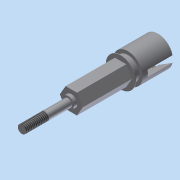
# Autodesk Inventor part: Shaft
Saved by Autodesk Inventor 2011 SP1 (Build 150282100, 282)
## iProperties
Created: 2011-09-20
Part Number: Shaft
Document SubType Name: Modeling
Designer: dgitz
Density: 1 g/cm^3
Author: dgitz
Autodesk Inventor part; units mm, degrees
ref_plane "YZ Plane" through (0, 0, 0) normal (1, 0, 0) x (0, 1, 0)
ref_plane "XZ Plane" through (0, 0, 0) normal (0, 1, 0) x (-1, 0, 0)
ref_plane "XY Plane" through (0, 0, 0) normal (0, 0, 1) x (1, 0, 0)
sketch "Sketch1" plane through (0, 0, 0) normal (0, 0, 1) x (1, 0, 0)
  line L0 (2.1997, -3.81) -> (-2.1997, -3.81)
  line L1 (-2.1997, -3.81) -> (-4.3994, 0)
  line L2 (-4.3994, 0) -> (-2.1997, 3.81)
  line L3 (-2.1997, 3.81) -> (2.1997, 3.81)
  line L4 (2.1997, 3.81) -> (4.3994, 0)
  line L5 (4.3994, 0) -> (2.1997, -3.81)
  point P0 (0, 0)
  point P1 (0, 0)
  dimension "d0" = 7.62
  constraints: 12 end point, 1 coincident, 1 horizontal, 13 other
  measures "d0" distance between parallel lines of L0 L3
extrude "Extrusion1" add sketch "Sketch1" along normal blind 19.05
sketch "Sketch2" plane through (0, 0, 19.05) normal (0, 0, 1) x (1, 0, 0)
  circle A0 centre (0, 0) radius 2.286
  dimension "d3" = 4.572
  constraints: 1 centre point, 1 coincident
  measures "d3" diameter of A0
extrude "Extrusion2" add sketch "Sketch2" along normal blind 1.27
sketch "Sketch3" plane through (0, 0, 20.32) normal (0, 0, 1) x (1, 0, 0)
  circle A0 centre (0, 0) radius 2.286 projected
  circle A1 centre (0, 0) radius 1.5875
  dimension "d6" = 3.175
  constraints: 1 centre point, 1 coincident
  measures "d6" diameter of A1
extrude "Extrusion3" add sketch "Sketch3" along normal blind 17.78 contours A1
thread "Thread1" size "5-40 UNC" class "2A" standard "ANSI Unified Screw Threads" length 8.89
sketch "Sketch4" plane through (0, 0, 0) normal (0, 0, -1) x (-1, 0, 0)
  circle A0 centre (0, 0) radius 5.715
  dimension "d11" = 11.43
  constraints: 1 centre point, 1 coincident
  measures "d11" diameter of A0
extrude "Extrusion4" add sketch "Sketch4" along normal blind 0.254
sketch "Sketch5" plane through (0, 0, -0.254) normal (0, 0, -1) x (-1, 0, 0)
  circle A0 centre (0, 0) radius 5.715 projected
  circle A1 centre (0, 0) radius 4.445
  dimension "d14" = 8.89
  constraints: 1 centre point, 1 coincident
  measures "d14" diameter of A1
extrude "Extrusion5" add sketch "Sketch5" along normal blind 2.54 contours A1
sketch "Sketch6" plane through (0, 0, -2.794) normal (0, 0, -1) x (-1, 0, 0)
  circle A0 centre (0, 0) radius 4.445 projected
  circle A1 centre (0, 0) radius 5.715
  dimension "d17" = 11.43
  constraints: 1 centre point, 1 coincident
  measures "d17" diameter of A1
extrude "Extrusion6" add sketch "Sketch6" along normal blind 2.032 contours A0 | A1
sketch "Sketch7" plane through (0, 0, -4.826) normal (0, 0, -1) x (-1, 0, 0)
  circle A0 centre (0, 0) radius 5.715 projected
  circle A1 centre (0, 0) radius 5.715 projected
  line L0 (0, 6.5237) -> (0, -6.5237) construction
  arc A2 (-3.5921, -1.27) -> (3.5921, -1.27) centre (0, 0) ccw
  arc A3 (3.5921, 1.27) -> (-3.5921, 1.27) centre (0, 0) ccw
  arc A4 (-5.5721, -1.27) -> (5.5721, -1.27) centre (0, 0) ccw
  arc A5 (5.5721, 1.27) -> (-5.5721, 1.27) centre (0, 0) ccw
  arc A6 (-3.5921, 1.27) -> (-3.5921, -1.27) centre (0, 0) ccw
  arc A7 (-5.5721, 1.27) -> (-5.5721, -1.27) centre (0, 0) ccw
  arc A8 (3.5921, -1.27) -> (3.5921, 1.27) centre (0, 0) ccw
  arc A9 (5.5721, -1.27) -> (5.5721, 1.27) centre (0, 0) ccw
  point P0 (-5.715, 1.27)
  point P1 (-5.715, -1.27)
  point P2 (5.715, 1.27)
  point P3 (5.715, -1.27)
  constraints: 16 point on circle, 8 centre point, 5 coincident, 4 symmetric about line, 2 end point, 1 midpoint
extrude "Extrusion8" add sketch "Sketch7" along normal blind 6.35
sketch "Sketch13" plane through (0, 0, 0) normal (1, 0, 0) x (0, 1, 0)
  line L0 (2.286, 20.32) -> (2.286, 19.05) projected
  line L1 (2.286, 19.05) -> (3.81, 19.05) projected
  line L2 (3.81, 19.05) -> (3.81, 0) projected
  line L3 (3.81, 0) -> (5.715, 0) projected
  line L4 (5.715, 0) -> (5.715, -0.254) projected
  line L5 (5.715, -0.254) -> (4.445, -0.254) projected
  line L6 (4.445, -0.254) -> (4.445, -2.794) projected
  line L7 (4.445, -2.794) -> (5.715, -2.794) projected
  line L8 (5.715, -2.794) -> (5.715, -11.176) projected
  line L9 (5.715, -11.176) -> (3.81, -11.176) projected
  line L10 (3.81, -11.176) -> (3.81, -4.826) projected
  line L11 (3.81, -4.826) -> (-3.81, -4.826) projected
  line L12 (-3.81, -4.826) -> (-3.81, -11.176) projected
  line L13 (-3.81, -11.176) -> (-5.715, -11.176) projected
  line L14 (-5.715, -11.176) -> (-5.715, -2.794) projected
  line L15 (-5.715, -2.794) -> (-4.445, -2.794) projected
  line L16 (-4.445, -2.794) -> (-4.445, -0.254) projected
  line L17 (-4.445, -0.254) -> (-5.715, -0.254) projected
  line L18 (-5.715, -0.254) -> (-5.715, 0) projected
  line L19 (-5.715, 0) -> (-3.81, 0) projected
  line L20 (-3.81, 0) -> (-3.81, 19.05) projected
  line L21 (-3.81, 19.05) -> (-2.286, 19.05) projected
  line L22 (-2.286, 19.05) -> (-2.286, 20.32) projected
  line L23 (-2.286, 20.32) -> (-1.5875, 20.32) projected
  line L24 (-1.5875, 20.32) -> (-1.5875, 38.1) projected
  line L25 (-1.5875, 38.1) -> (1.5875, 38.1) projected
  line L26 (1.5875, 38.1) -> (1.5875, 20.32) projected
  line L27 (1.5875, 20.32) -> (2.286, 20.32) projected
  line L28 (5.715, -11.176) -> (5.715, -14.4756)
  line L29 (5.715, -14.4756) -> (3.81, -11.176)
  line L30 (3.81, -11.176) -> (5.715, -11.176)
  line L31 (0, -24.9907) -> (0, 48.6151) projected
  point P0 (0, 0)
  dimension "d32" = 30
  constraints: 6 end point, 1 vertical
  measures "d32" angle of L29 L28
revolve "Revolution1" add sketch "Sketch13" angle 360 about axis through (0, 0, -10) along (0, 0, 1) contours L9 L28 L29
sketch "Sketch16" plane through (0, 0, -4.826) normal (0, 0, -1) x (-1, 0, 0)
  circle A0 centre (0, 0) radius 3.81 projected
  line L0 (-5.5721, 1.27) -> (-3.5921, 1.27)
  line L1 (-3.5921, -1.27) -> (-5.5721, -1.27)
  arc A1 (-3.5921, 1.27) -> (-3.5921, -1.27) centre (0, 0) ccw
  arc A2 (-5.5721, 1.27) -> (-5.5721, -1.27) centre (0, 0) ccw
  circle A3 centre (0, 0) radius 5.715 projected
  line L2 (5.5721, -1.27) -> (3.5921, -1.27)
  line L3 (3.5921, 1.27) -> (5.5721, 1.27)
  arc A4 (3.5921, -1.27) -> (3.5921, 1.27) centre (0, 0) ccw
  arc A5 (5.5721, -1.27) -> (5.5721, 1.27) centre (0, 0) ccw
  dimension "d47" = 360
  constraints: 12 point on circle, 8 end point, 4 centre point, 3 coincident, 2 concentric, 1 horizontal, 1 parallel, 21 other
extrude "Extrusion9" cut sketch "Sketch16" along normal up to surface contours A0 L3 A3 L2 | A0 L1 A2 L0
body "Solid1"
